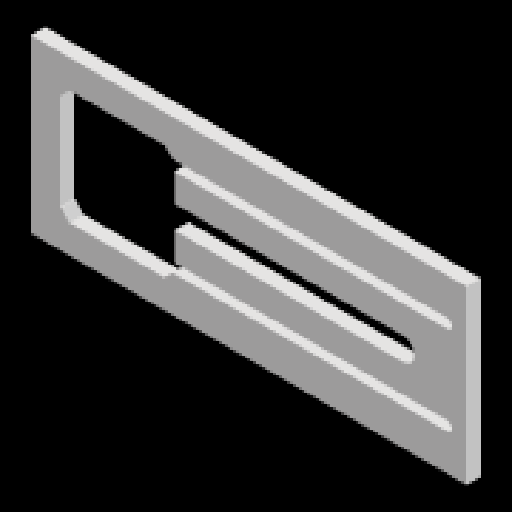
# Autodesk Inventor part: CombineTestHorizontal
Saved by Autodesk Inventor 2025 (Build 290162000, 162)
## iProperties
Created: 2025-01-20
Part Number: CombineTestHorizontal
Material: Generic
Document SubType Name: Modeling
Designer: Trevor
Density: 1 g/cm^3
Appearance: Default
Author: Trevor
Autodesk Inventor part; units mm, degrees
ref_plane "YZ Plane" through (0, 0, 0) normal (1, 0, 0) x (0, 1, 0)
ref_plane "XZ Plane" through (0, 0, 0) normal (0, 1, 0) x (-1, 0, 0)
ref_plane "XY Plane" through (0, 0, 0) normal (0, 0, 1) x (1, 0, 0)
sketch "Sketch1" plane through (0, 0, 0) normal (0, 0, 1) x (1, 0, 0)
  line L0 (-20, 16.5858) -> (-16.5858, 20) projected
  line L1 (-20, -16.5858) -> (-20, 16.5858) projected
  line L2 (-16.5858, -20) -> (-20, -16.5858) projected
  line L3 (16.5858, -20) -> (-16.5858, -20) projected
  line L4 (20, -16.5858) -> (16.5858, -20) projected
  line L5 (20, 16.5858) -> (20, -16.5858) projected
  line L6 (16.5858, 20) -> (20, 16.5858) projected
  line L7 (-16.5858, 20) -> (16.5858, 20) projected
  circle A0 centre (15.5, -15.5) radius 1.5 projected
  circle A1 centre (-15.5, 15.5) radius 1.5 projected
  circle A2 centre (-15.5, -15.5) radius 1.5 projected
  circle A3 centre (15.5, 15.5) radius 1.5 projected
  circle A4 centre (0, 0) radius 11 projected
  line L8 (-20, 0) -> (-30, 0) construction
  line L9 (-20, 0) -> (-20, -30)
  line L10 (-20, -30) -> (-30, -30)
  line L11 (-30, -30) -> (-30, 30)
  line L12 (-30, 30) -> (-20, 30)
  line L13 (-20, 30) -> (-20, -30)
  line L14 (-15.5, -17) -> (-20, -17)
  line L15 (-20, 17) -> (-15.5, 17)
  line L16 (0, 0) -> (100, 0.0668) construction
  circle A5 centre (0, 0) radius 3.8 construction
  circle A6 centre (0, 0) radius 4 construction
  line L17 (0, 0) -> (100, 0.0668) construction
  line L18 (0.0027, -4) -> (100.0026, -3.9332)
  line L19 (99.9973, 4.0668) -> (-0.0027, 4)
  arc A7 (-0.0027, 4) -> (0.0027, -4) centre (0, 0) ccw
  arc A8 (100.0026, -3.9332) -> (99.9973, 4.0668) centre (100, 0.0668) ccw
  line L20 (15.5, -15.5) -> (0, -15.5) construction
  line L21 (15.5, -15.5) -> (115.5, -15.5) construction
  line L22 (15.5, 15.5) -> (115.5, 15.5) construction
  line L23 (115.5, 15.5) -> (115.5, -15.5) construction
  circle A9 centre (-15.5, -15.5) radius 1.7 construction
  circle A10 centre (-15.5, 15.5) radius 1.7 construction
  line L24 (-15.5, 15.5) -> (115.5, 15.5) construction
  line L25 (-15.5, 17.2) -> (115.5, 17.2)
  line L26 (115.5, 13.8) -> (-15.5, 13.8)
  arc A11 (-15.5, 17.2) -> (-15.5, 13.8) centre (-15.5, 15.5) ccw
  arc A12 (115.5, 13.8) -> (115.5, 17.2) centre (115.5, 15.5) ccw
  line L27 (-15.5, -15.5) -> (115.5, -15.5) construction
  line L28 (-15.5, -13.8) -> (115.5, -13.8)
  line L29 (115.5, -17.2) -> (-15.5, -17.2)
  arc A13 (-15.5, -13.8) -> (-15.5, -17.2) centre (-15.5, -15.5) ccw
  arc A14 (115.5, -17.2) -> (115.5, -13.8) centre (115.5, -15.5) ccw
  line L30 (117.2, 15.5) -> (122.2, 15.5) construction
  line L31 (-20, 30) -> (122.2, 30)
  line L32 (122.2, 30) -> (122.2, -30)
  line L33 (122.2, -30) -> (-20, -30)
  point P0 (50, 0.0334)
  point P1 (50, 15.5)
  point P2 (50, -15.5)
  point P3 (-19.5858, 17)
  point P4 (19.3858, 17.2)
  point P5 (20, 13.8)
  point P6 (20, 4.0134)
  point P7 (20, -3.9866)
  point P8 (20, -13.8)
  point P9 (19.3858, -17.2)
  point P10 (-19.5858, -17)
  point P11 (-16.3, 17)
  dimension "d0" = 10
  dimension "d1" = 30
  dimension "d2" = 10
  dimension "d3" = 60
  dimension "d6" = 100
  dimension "d7" = 0.2
  dimension "d8" = 100
  dimension "d9" = 0.2
  dimension "d10" = 0.2
  dimension "d11" = 5
  constraints: 58 end point, 13 point on circle, 12 tangent, 9 centre point, 9 horizontal, 6 parallel, 5 perpendicular, 4 midpoint, 3 concentric, 2 collinear, 2 point on line, 2 vertical alignment, 1 vertical, 2 other
  measures "d0" distance of L8.start L8.end
  measures "d1" distance of L8.start L9.end
  measures "d2" distance of L11.end L12.end
  measures "d3" distance of L10.end L11.end
  measures "d6" distance of L16.start L16.end
  measures "d7" radial gap between concentric circles of A5 A6
  measures "d8" distance of L20.start L21.end
  measures "d11" distance of L30.start L30.end
extrude "Extrusion1" add sketch "Sketch1" along normal blind 5 contours L0 L15 A11 L26 L5 L19 A4 L18 L28 A13 L14 L2 L1 | L1 L9 L10 L11 L12 L13 | L15 L13 L31 L32 L33 L9 L14 L2 L3 L4 L29 A14 L28 L5 L18 A8 L19 L26 A12 L25 L6 L7 L0 | L0 L7 L6 L25 A11 L15 | L14 A13 L29 L4 L3 L2 | L19 A7 L18 A4 picked at (6.4115, 4.7804)
sketch "Sketch2" plane through (-30, -30, 0) normal (-1, 0, 0) x (0, 0, 1)
  point P0 (0, 30)
sketch "Sketch3" plane through (-30, -30, 0) normal (-1, 0, 0) x (0, 0, 1)
  line L0 (0, 60) -> (0, 0) projected
  line L1 (0, 0) -> (5, 0) projected
  line L2 (5, 60) -> (5, 0) projected
  line L3 (0, 60) -> (5, 60) projected
  line L4 (10, -5) -> (-5, -5)
  line L5 (-5, -5) -> (-5, 65)
  line L6 (-5, 65) -> (10, 65)
  line L7 (10, 65) -> (10, -5)
  line L8 (0, 47.2) -> (0, 43.8) projected
  line L9 (-0.7217, 45.5) -> (5, 45.5)
  circle A0 centre (2.1391, 45.5) radius 1.5
  point P0 (0, 30)
  point P1 (-1.5323, 14.5)
  dimension "d15" = 5
  dimension "d16" = 3
  constraints: 10 end point, 1 centre point, 1 midpoint, 1 perpendicular, 1 point on line, 3 other
  measures "d15" distance between parallel lines of L2 L7
  measures "d16" diameter of A0
body "Solid1"
